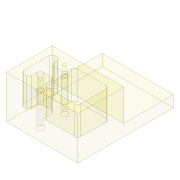
# Autodesk Inventor part: zgalvo_cover
Saved by Autodesk Inventor 2018.2 (Build 222227000, 227)
## iProperties
Created: 2018-07-24
Part Number: zgalvo_cover
Material: Generic
Document SubType Name: Modeling
Designer: LegantLab
Density: 1 g/cm^3
Appearance: Clear - Yellow
Catalog Web Link: https://www.shapeways.com
Author: LegantLab
Autodesk Inventor part; units mm, degrees
ref_plane "YZ Plane" through (0, 0, 0) normal (1, 0, 0) x (0, 1, 0)
ref_plane "XZ Plane" through (0, 0, 0) normal (0, 1, 0) x (-1, 0, 0)
ref_plane "XY Plane" through (0, 0, 0) normal (0, 0, 1) x (1, 0, 0)
sketch "Sketch1" plane through (0, 0, 0) normal (0, 0, 1) x (1, 0, 0)
  line L0 (-17.5, 16) -> (17.5, 16)
  line L1 (17.5, 16) -> (17.5, -16)
  line L2 (17.5, -16) -> (-17.5, -16)
  line L3 (-17.5, -16) -> (-17.5, 16)
  point P0 (0, 0)
  dimension "d0" = 35
  dimension "d1" = 32
  dimension "d2" = 16
  dimension "d3" = 17.5
  constraints: 8 end point, 2 parallel, 1 horizontal, 1 perpendicular
  measures "d0" distance of L1.end L2.end
  measures "d1" distance of L2.end L0.start
  measures "d2" distance from line of L0 point (0, 0)
  measures "d3" distance from line of L1 point (0, 0)
extrude "Extrusion1" add sketch "Sketch1" along normal blind 30
sketch "Sketch2" plane through (-17.5, 16, 0) normal (0, 1, 0) x (1, 0, 0)
  line L0 (0, 0) -> (35, 0) projected
  line L1 (0, 0) -> (0, -30) projected
  line L2 (35, -30) -> (0, -30) projected
  line L3 (35, 0) -> (35, -30) projected
  line L4 (0, 0) -> (0, -30) projected
  line L5 (35, 0) -> (35, -30) projected
  line L6 (0, 0) -> (35, 0)
  line L7 (35, 0) -> (35, -8)
  line L8 (35, -8) -> (0, -8)
  line L9 (0, -8) -> (0, 0)
  point P0 (17.5, 0)
  dimension "d6" = 8
  constraints: 8 end point, 2 parallel, 1 horizontal, 1 perpendicular, 1 point on line
  measures "d6" distance between parallel lines of L0 L8
extrude "Extrusion2" add sketch "Sketch2" along normal blind 35 contours L0 L3 L8 L1
sketch "Sketch3" plane through (0, 0, 0) normal (0, 0, -1) x (-1, 0, 0)
  circle A0 centre (1.75, -8) radius 0.7835 projected
  circle A1 centre (1.75, 9) radius 0.7835 projected
  point P0 (0, 0)
hole "Hole1" at (-1.75, 9, 0) at (-1.75, -8, 0) direction (0, 0, 1) diameter 2.4 end through all counterbore diameter 4.4 counterbore depth 23 clearance for "Socket Head Cap Screw" size "M2" standard "Ansi Metric M Profile"
sketch "Sketch4" plane through (17.5, -16, 30) normal (1, 0, 0) x (0, 0, -1)
  line L0 (30, 67) -> (30, 0) projected
  line L1 (22, 67) -> (30, 67) projected
  line L2 (22, 32) -> (22, 67) projected
  line L3 (22, 32) -> (0, 32) projected
  line L4 (0, 0) -> (0, 32) projected
  line L5 (30, 0) -> (0, 0) projected
  point P0 (30, 16)
extrude "Extrusion3" add sketch "Sketch4" along normal blind 15
sketch "Sketch7" plane through (0, 0, 30) normal (0, 0, 1) x (1, 0, 0)
  circle A0 centre (-1.75, 9) radius 1.2 projected
  circle A1 centre (-1.75, -8) radius 1.2 projected
  line L0 (-17.5, 16) -> (32.5, 16) projected
  line L1 (-17.5, 16) -> (-17.5, -16) projected
  line L2 (-17.5, -16) -> (32.5, -16) projected
  line L3 (32.5, 16) -> (32.5, -16) projected
  line L4 (-6.75, -9) -> (-6.75, -5)
  line L5 (-4.75, -3) -> (1.25, -3)
  line L6 (3.25, -5) -> (3.25, -9)
  line L7 (5.25, -11) -> (25.5, -11)
  line L8 (27.5, -9) -> (27.5, 9)
  line L9 (25.5, 11) -> (5.25, 11)
  line L10 (3.25, 9) -> (3.25, 6)
  line L11 (1.25, 4) -> (-4.75, 4)
  line L12 (-6.75, 6) -> (-6.75, 9)
  line L13 (-8.75, 11) -> (-10.5, 11)
  line L14 (-12.5, 9) -> (-12.5, -9)
  line L15 (-10.5, -11) -> (-8.75, -11)
  arc A2 (-4.75, -3) -> (-6.75, -5) centre (-4.75, -5) ccw
  arc A3 (-8.75, -11) -> (-6.75, -9) centre (-8.75, -9) ccw
  arc A4 (-12.5, -9) -> (-10.5, -11) centre (-10.5, -9) ccw
  arc A5 (-10.5, 11) -> (-12.5, 9) centre (-10.5, 9) ccw
  arc A6 (-6.75, 9) -> (-8.75, 11) centre (-8.75, 9) ccw
  arc A7 (-6.75, 6) -> (-4.75, 4) centre (-4.75, 6) ccw
  arc A8 (1.25, 4) -> (3.25, 6) centre (1.25, 6) ccw
  arc A9 (5.25, 11) -> (3.25, 9) centre (5.25, 9) ccw
  arc A10 (27.5, 9) -> (25.5, 11) centre (25.5, 9) ccw
  arc A11 (25.5, -11) -> (27.5, -9) centre (25.5, -9) ccw
  arc A12 (3.25, -9) -> (5.25, -11) centre (5.25, -9) ccw
  arc A13 (3.25, -5) -> (1.25, -3) centre (1.25, -5) ccw
  point P0 (0, 0)
  point P1 (3.25, 11)
  point P2 (3.25, 4)
  point P3 (-6.75, 4)
  point P4 (-6.75, 11)
  point P5 (-12.5, -11)
  dimension "d18" = 5
  dimension "d19" = 5
  dimension "d21" = 5
  dimension "d22" = 5
  dimension "d23" = 5
  dimension "d24" = 5
  dimension "d25" = 5
  dimension "d26" = 5
  dimension "d27" = 5
  dimension "d28" = 2
  dimension "d29" = 2
  constraints: 24 end point, 24 point on circle, 24 tangent, 15 point on line, 12 centre point, 10 equal radius, 9 perpendicular, 1 vertical
  measures "d18" distance between parallel lines of L1 L14
  measures "d19" distance between parallel lines of L3 L8
  measures "d21" distance from line of A1.centre L4
  measures "d22" distance from line of L6 A1.centre
  measures "d23" distance between parallel lines of L2 L7
  measures "d24" distance between parallel lines of L0 L9
  measures "d25" distance between parallel lines of L0 L13
  measures "d26" distance from line of A0.centre L11
  measures "d27" distance from line of L5 A1.centre
  measures "d28" radius of A2
  measures "d29" radius of A13
extrude "Extrusion4" cut sketch "Sketch7" against normal blind 20 contours A3 L15 A4 L14 A5 L13 A6 L12 A7 L11 A8 L10 A9 L9 A10 L8 A11 L7 A12 L6 A13 L5 A2 L4
equation "\"d2\" = 0.5 * d1"
equation "\"d3\" = 0.5 * d0"
body "Solid1"
